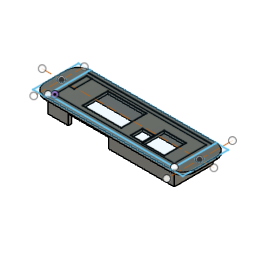
Temperaturos_valdiklis v11 (Autodesk Fusion 360 design; units mm, degrees)
Autodesk Fusion 360 part; units mm, degrees
sketch "Sketch1" plane through (0, 0, 0) normal (0, 0, 1) x (1, 0, 0)
  line L0 (0, 0) -> (71, 0)
  line L1 (71, 0) -> (71, 19)
  line L2 (71, 19) -> (0, 19)
  line L3 (0, 19) -> (0, 0)
  line L4 (14, 17.5) -> (37, 17.5)
  line L5 (37, 17.5) -> (37, 2.5)
  line L6 (37, 2.5) -> (14, 2.5)
  line L7 (14, 2.5) -> (14, 17.5)
  line L8 (-2, 21) -> (73, 21)
  line L9 (73, -2) -> (-2, -2)
  line L10 (51, 14) -> (64, 14)
  line L11 (64, 14) -> (64, 1)
  line L12 (64, 1) -> (51, 1)
  line L13 (51, 1) -> (51, 14)
  line L14 (43.6, 8.5) -> (50.6, 8.5)
  line L15 (50.6, 8.5) -> (50.6, 1.5)
  line L16 (50.6, 1.5) -> (43.6, 1.5)
  line L17 (43.6, 1.5) -> (43.6, 8.5)
  line L18 (73, -2) -> (73, 21)
  line L19 (-2, -2) -> (-2, 21)
  line L20 (-17.0313, 9.5) -> (85, 9.5) construction
  line L21 (-5.5, 23) -> (-5.5, -7) construction
  circle A0 centre (-5.5, 9.5) radius 1.75
  line L22 (76.5, 29) -> (76.5, -10) construction
  circle A1 centre (76.5, 9.5) radius 1.75
  line L23 (-2, 23) -> (-9, 23)
  line L24 (-9, 23) -> (-9, -3.9661)
  line L25 (-9, -3.9661) -> (-2, -3.9661)
  line L26 (-2, -3.9661) -> (-2, 23)
  line L27 (73, 23) -> (80, 23)
  line L28 (80, 23) -> (80, -4)
  line L29 (80, -4) -> (73, -4)
  line L30 (73, -4) -> (73, 23)
  line L31 (-2, 23) -> (73, 23)
  line L32 (73, 23) -> (73, 21)
  line L33 (73, 21) -> (-2, 21)
  line L34 (-2, 21) -> (-2, 23)
  line L35 (-2, -2) -> (73, -2)
  line L36 (73, -2) -> (73, -4)
  line L37 (73, -4) -> (-2, -4)
  line L38 (-2, -4) -> (-2, -2)
  line L39 (0, 19) -> (3, 19)
  line L40 (3, 19) -> (3, 8.5)
  line L41 (3, 8.5) -> (0, 8.5)
  line L42 (0, 8.5) -> (0, 19)
  dimension "d2" = 71
  dimension "d3" = 19
  dimension "d6" = 23
  dimension "d7" = 15
  dimension "d8" = 14
  dimension "d9" = 1.5
  dimension "d16" = 75
  dimension "d17" = 23
  dimension "d18" = 2
  dimension "d32" = 13
  dimension "d33" = 13
  dimension "d34" = 20
  dimension "d35" = 14
  dimension "d36" = 7
  dimension "d37" = 7
  dimension "d38" = 27.4
  dimension "d39" = 8.5
  dimension "d61" = 3.5
  dimension "d63" = 3.5
  dimension "d70" = 7
  dimension "d79" = 10.5
  dimension "d80" = 3
  constraint horizontal L0
  constraint vertical L1
  constraint horizontal L2
  constraint vertical L3
  constraint coincident L0.start L3.end
  constraint horizontal L4
  constraint vertical L5
  constraint horizontal L6
  constraint vertical L7
  constraint horizontal L8
  constraint horizontal L9
  constraint horizontal L10
  constraint vertical L11
  constraint horizontal L12
  constraint vertical L13
  constraint horizontal L14
  constraint vertical L15
  constraint horizontal L16
  constraint vertical L17
  constraint vertical L18
  constraint vertical L19
  constraint coincident L20 A0.centre
  constraint coincident L21 A0.centre
  constraint midpoint L22 A1.centre
  constraint horizontal L23
  constraint vertical L24
  constraint horizontal L25
  constraint vertical L26
  constraint horizontal L27
  constraint vertical L28
  constraint horizontal L29
  constraint vertical L30
  constraint horizontal L31
  constraint vertical L32
  constraint horizontal L33
  constraint vertical L34
  constraint horizontal L35
  constraint vertical L36
  constraint horizontal L37
  constraint vertical L38
  constraint horizontal L39
  constraint vertical L40
  constraint horizontal L41
  constraint vertical L42
  measures "d2" distance of L0.start L0.end
  measures "d3" distance of L0.start L2.end
  measures "d6" distance of L4.start L4.end
  measures "d7" distance of L4.start L6.end
  measures "d8" distance of L3 L7
  measures "d9" distance of L2 L4
  measures "d16" distance of L8.start L8.end
  measures "d17" distance of L8.start L9.end
  measures "d18" distance of L2 L8
  measures "d32" distance of L10.start L10.end
  measures "d33" distance of L10.start L12.end
  measures "d34" distance of L1 L13
  measures "d35" distance of L0 L10
  measures "d36" distance of L14.start L14.end
  measures "d37" distance of L14.start L16.end
  measures "d38" distance of L1 L17
  measures "d39" distance of L0 L14
  measures "d61" diameter of A0
  measures "d63" diameter of A1
  measures "d70" distance of L19 L24
  measures "d79" distance of L2 L41
  measures "d80" distance of L3 L40
extrude "Extrude2" add sketch "Sketch1" against normal blind 10 contours L8 L9 L18 L19 L26 L30 L33 L35
extrude "Extrude3" add sketch "Sketch1" against normal blind 1.5 contours L0 L1 L2 L3 L40 L41 | L2 L3 L39 L40 L41 L42 | L10 L11 L12 L13 | L14 L15 L16 L17
sketch "Sketch3" plane through (73, 0, 0) normal (1, 0, 0) x (0, 1, 0)
  line L0 (21, 0) -> (-2, 0)
  line L1 (-2, 0) -> (-2, -10)
  line L2 (-2, -10) -> (21, -10)
  line L3 (21, -10) -> (21, 0)
  line L4 (0.0991, -10) -> (10.0991, -10)
  line L5 (10.0991, -10) -> (10.0991, -2)
  line L6 (10.0991, -2) -> (0.0991, -2)
  line L7 (0.0991, -2) -> (0.0991, -10)
  dimension "d24" = 10
  dimension "d25" = 8
  constraint horizontal L4
  constraint vertical L5
  constraint horizontal L6
  constraint vertical L7
  constraint coincident L2 L4.start
  measures "d24" distance of L4.start L4.end
  measures "d25" distance of L4.start L6.end
sketch "Sketch4" plane through (-2, 0, 0) normal (-1, 0, 0) x (0, -1, 0)
  line L0 (2, 0) -> (-21, 0)
  line L1 (-21, 0) -> (-21, -10)
  line L2 (-21, -10) -> (2, -10)
  line L3 (2, -10) -> (2, 0)
  line L4 (-0.0261, -10) -> (-8.0261, -10)
  line L5 (-8.0261, -10) -> (-8.0261, -2)
  line L6 (-8.0261, -2) -> (-0.0261, -2)
  line L7 (-0.0261, -2) -> (-0.0261, -10)
  dimension "d28" = 8
  dimension "d29" = 8
  constraint horizontal L4
  constraint vertical L5
  constraint horizontal L6
  constraint vertical L7
  constraint coincident L2 L4.start
  measures "d28" distance of L4.start L4.end
  measures "d29" distance of L4.start L6.end
extrude "Extrude6" cut sketch "Sketch1" against normal blind 3 contours L14 L15 L16 L17
extrude "Extrude7" cut sketch "Sketch1" against normal blind 3 contours L10 L11 L12 L13
sketch "Sketch5" plane through (0, -2, 0) normal (0, -1, 0) x (1, 0, 0)
  line L0 (73, 0) -> (-2, 0)
  line L1 (-2, -10) -> (73, -10)
  line L2 (10, -4) -> (34, -4)
  line L3 (34, -4) -> (34, -10)
  line L4 (34, -10) -> (10, -10)
  line L5 (10, -10) -> (10, -4)
  line L6 (73, 0) -> (-2, 0)
  line L7 (-2, 0) -> (-2, -10)
  line L8 (73, -10) -> (73, 0)
  dimension "d44" = 4
  dimension "d45" = 10
  dimension "d46" = 24
  dimension "d47" = 6
  constraint horizontal L2
  constraint vertical L3
  constraint horizontal L4
  constraint vertical L5
  measures "d44" distance of L2 L6
  measures "d45" distance of L5 origin
  measures "d46" distance of L3 L5
  measures "d47" distance of L2 L4
extrude "Extrude8" cut sketch "Sketch5" against normal blind 3 contours L1 L2 L3 L4 L5
extrude "Extrude10" cut sketch "Sketch1" against normal blind 4 contours A0
extrude "Extrude11" cut sketch "Sketch1" against normal blind 4 contours A1
extrude "Extrude12" add sketch "Sketch1" against normal blind 1.5 contours L8 L26 L30 L31 L32 L33 L34 | L9 L26 L30 L35 L36 L37 L38
sketch "Sketch2" plane through (0, 0, 0) normal (0, 0, 1) x (1, 0, 0)
extrude "Extrude13" add sketch "Sketch1" against normal blind 1.5 contours L19 L23 L24 L25 L26 L34 L38 | L18 L27 L28 L29 L30 L32 L36
fillet "Fillet2" radius 7 4 edges at (-9, -3.9661, -0.75) (80, 23, -0.75) (80, -4, -0.75) (-9, 23, -0.75)
extrude "Extrude14" add sketch "Sketch1" against normal blind 7 contours L2 L3 L39 L40 L41 L42
